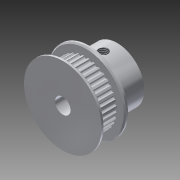
# Autodesk Inventor part: PulleyGT2x32x5Bore
Saved by Autodesk Inventor 2015 SP1 (Build 190203100, 203)
## iProperties
Category: Hardware
Created: 2014-08-25
Part Number: PulleyGT2x32x5Bore
Material: Aluminum 6061
Document SubType Name: Modeling
Designer: t_clevj
Density: 2.7 g/cm^3
Appearance: Aluminum - Flat
Mass: 12.3426 g
Surface Area: 28.859 cm^2
Volume: 4.57135 cm^3
Vendor: Misumi
Catalog Web Link: http://us.misumi-ec.com/vona2/detail/110302193470
Stock Number: GPA36GT2060-B-H8
Author: Jack
Title: Pulley GT2 36T 5mm Bore
Autodesk Inventor part; units mm, degrees
ref_plane "XZ Plane" through (0, 0, 0) normal (0, 1, 0) x (-1, 0, 0)
sketch "Sketch1" plane through (0, 0, 0) normal (0, 1, 0) x (-1, 0, 0)
  circle A0 centre (0, 0) radius 12.5
  dimension "d0" = 25
  constraints: 1 centre point, 1 coincident
  measures "d0" diameter of A0
extrude "Extrusion1" add sketch "Sketch1" along normal blind 1
chamfer "Chamfer1" distance 0.4 angle 45 1 edges at (12.5, 1, 0)
sketch "Sketch2" plane through (0, 1, 0) normal (0, 1, 0) x (1, 0, 0)
  circle A0 centre (0, 0) radius 12.1 projected
  circle A1 centre (0, 0) radius 9.9
  dimension "d6" = 19.8
  constraints: 1 centre point, 1 coincident
  measures "d6" diameter of A1
extrude "Extrusion2" add sketch "Sketch2" along normal blind 6.5 contours A1
sketch "Sketch3" plane through (0, 7.5, 0) normal (0, 1, 0) x (1, 0, 0)
  circle A0 centre (0, 0) radius 12.5 projected
extrude "Extrusion3" add sketch "Sketch3" along normal blind 1
sketch "Sketch4" plane through (0, 8.5, 0) normal (0, 1, 0) x (1, 0, 0)
  circle A0 centre (0, 0) radius 8.75
  dimension "d14" = 17.5
  constraints: 1 centre point, 1 coincident
  measures "d14" diameter of A0
extrude "Extrusion4" add sketch "Sketch4" along normal blind 9
sketch "Sketch5" plane through (0, 17.5, 0) normal (0, 1, 0) x (1, 0, 0)
  circle A0 centre (0, 0) radius 8.75 projected
  circle A1 centre (0, 0) radius 2.5
  dimension "d17" = 5
  constraints: 1 centre point, 1 coincident
  measures "d17" diameter of A1
extrude "Extrusion5" cut sketch "Sketch5" against normal up to surface (17.5 mm away) contours A1
sketch "Sketch6" plane through (0, 1, 0) normal (0, 1, 0) x (1, 0, 0)
  circle A0 centre (0, 0) radius 9.9 projected
  arc A1 (0.5997, -9.8818) -> (-0.5997, -9.8818) centre (0, -9.9) ccw
  dimension "d20" = 1.2
  constraints: 5 point on circle, 1 centre point, 1 vertical alignment
  measures "d20" diameter of A1
extrude "Extrusion6" cut sketch "Sketch6" along normal up to surface (6.5 mm away) contours A1 A0 picked at (-0.0236, -9.7001)
pattern_circular "Circular Pattern1" count 36 over 360 about axis through (0, 1, 0) along (0, 1, 0) of "Extrusion6"
ref_plane "Work Plane1" through (0, 0, 9) normal (0, 0, 1) x (1, 0, 0)
ref_plane "Work Plane2" through (-9, 0, 0) normal (1, 0, 0) x (0, 1, 0)
sketch "Sketch7" plane through (-9, 0, 0) normal (1, 0, 0) x (0, 1, 0)
  circle A0 centre (13, 0) radius 1.5
  line L0 (17.5, -8.75) -> (17.5, 8.75) projected
  point P0 (0, 0)
  dimension "d28" = 3
  dimension "d29" = 4.5
  constraints: 1 centre point, 1 horizontal alignment
  measures "d28" diameter of A0
  measures "d29" distance from line of L0 A0.centre
extrude "Extrusion7" cut sketch "Sketch7" along normal blind 7.25
sketch "Sketch8" plane through (0, 0, 9) normal (0, 0, 1) x (1, 0, 0)
  circle A0 centre (0, 13) radius 1.5
  line L0 (12.5, 8.5) -> (-12.5, 8.5) projected
  point P0 (0, 0)
  dimension "d32" = 3
  dimension "d40" = 4.5
  constraints: 1 centre point, 1 vertical alignment
  measures "d32" diameter of A0
  measures "d40" distance from line of L0 A0.centre
extrude "Extrusion8" cut sketch "Sketch8" against normal blind 8
thread "Thread1" size "M3x0.5" class "6H" standard "ANSI Metric M Profile" full length
thread "Thread2" size "M3x0.5" class "6H" standard "ANSI Metric M Profile" full length
chamfer "Chamfer3" distance 0.4 angle 45 1 edges at (-12.5, 7.5, 0)
body "Solid1"
